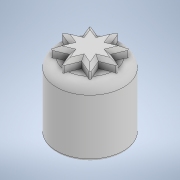
# Autodesk Inventor part: Button_Cap
Saved by Autodesk Inventor 2020 (Build 240168000, 168)
## iProperties
Created: 2020-05-25
Part Number: Button_Cap
Material: Generic
Document SubType Name: Modeling
Designer: maple
Density: 1 g/cm^3
Appearance: Default
Author: maple
Autodesk Inventor part; units mm, degrees
ref_plane "YZ Plane" through (0, 0, 0) normal (1, 0, 0) x (0, 1, 0)
ref_plane "XZ Plane" through (0, 0, 0) normal (0, 1, 0) x (-1, 0, 0)
ref_plane "XY Plane" through (0, 0, 0) normal (0, 0, 1) x (1, 0, 0)
sketch "Sketch1" plane through (0, 0, 0) normal (0, 1, 0) x (-1, 0, 0)
  circle A0 centre (0, 0) radius 3.5
  circle A1 centre (0, 0) radius 7
  circle A2 centre (0, 0) radius 4.5
  circle A3 centre (0, 0) radius 6
  dimension "d0" = 7
  dimension "d1" = 14
  dimension "d2" = 9
  dimension "d3" = 12
  constraints: 4 centre point, 4 coincident
  measures "d0" diameter of A0
  measures "d1" diameter of A1
  measures "d2" diameter of A2
  measures "d3" diameter of A3
extrude "Extrusion1" add sketch "Sketch1" along normal blind 12
sketch "Sketch2" plane through (0, 12, 0) normal (0, 1, 0) x (1, 0, 0)
  circle A0 centre (0, 0) radius 7
  dimension "d6" = 14
  constraints: 1 centre point, 1 coincident
  measures "d6" diameter of A0
extrude "Extrusion2" add sketch "Sketch2" along normal blind 2
sketch "Sketch3" plane through (0, 12, 0) normal (0, -1, 0) x (1, 0, 0)
  circle A0 centre (0, 0) radius 3.5
  constraints: 1 centre point, 1 coincident
extrude "Extrusion3" add sketch "Sketch3" along normal blind 9
fillet "Fillet1" radius 0.5 4 edges at (4.5, 0, 0) (3.5, 0, 0) (7, 0, 0) (6, 0, 0)
sketch "Sketch4" plane through (0, 14, 0) normal (0, 1, 0) x (1, 0, 0)
  circle A0 centre (0, 0) radius 3.5
  circle A1 centre (0, 0) radius 6
  line L0 (0, -6) -> (-4.242641, 4.242641)
  line L1 (0, -6) -> (4.242641, 4.242641)
  line L2 (4.242641, -4.242641) -> (-6, 0)
  line L3 (4.242641, -4.242641) -> (0, 6)
  line L4 (6, 0) -> (-4.242641, -4.242641)
  line L5 (6, 0) -> (-4.242641, 4.242641)
  line L6 (-4.242641, -4.242641) -> (0, 6)
  line L7 (4.242641, 4.242641) -> (-6, 0)
  point P0 (3, -1.242641)
  point P1 (3, 1.242641)
  point P2 (1.242641, 3)
  point P3 (-1.242641, 3)
  point P4 (-3, 1.242641)
  point P5 (-3, -1.242641)
  point P6 (-1.242641, -3)
  point P7 (1.242641, -3)
  dimension "d14" = 360
  constraints: 16 end point, 1 perpendicular, 1 vertical alignment, 10 other
extrude "Extrusion4" add sketch "Sketch4" along normal blind 2 contours A0 L4 L3 L1 L5 | A0 L5 L4 | L1 L5 L3 L7 A0 | A0 L7 L1 | L1 L3 L5 | L3 L2 A0 | A0 L2 L1 L4 L3 | L4 L1 L3 | L1 L4 L2 L0 L6 L7 L5 L3 | L5 L7 L3 | L1 L2 L4 | L3 L7 L5 L6 A0 | A0 L6 L3 | L0 A0 L1 | L7 L6 L5 | A0 L0 L4 L2 L1 | L4 L0 L2 | L5 A0 L0 | L6 A0 L4 | L6 L7 L0 A0 L5 | L6 L0 L7 | L2 L6 L0 | L0 L4 A0 L6 L2 | L7 A0 L2 | L6 L2 A0 L7 L0
chamfer "Chamfer1" distance 0.7 angle 45 16 edges at (2.7426, 16, -3.6213) (3.6213, 16, -2.7426) (4.5, 16, -0.6213) (4.5, 16, 0.6213) (3.6213, 16, 2.7426) (2.7426, 16, 3.6213) (0.6213, 16, 4.5) (-0.6213, 16, 4.5) (-2.7426, 16, 3.6213) (-3.6213, 16, 2.7426) (-4.5, 16, 0.6213) (-4.5, 16, -0.6213) (-3.6213, 16, -2.7426) (-2.7426, 16, -3.6213) (-0.6213, 16, -4.5) (0.6213, 16, -4.5)
fillet "Fillet2" radius 2 1 edges at (-7, 14, 0)
fillet "Fillet3" radius 0.2 8 edges at (4.2426, 14.516, -4.2426) (0, 14.516, -6) (-4.2426, 14.516, -4.2426) (-6, 14.516, 0) (-4.2426, 14.516, 4.2426) (6, 14.516, 0) (4.2426, 14.516, 4.2426) (0, 14.516, 6)
body "Solid1"
